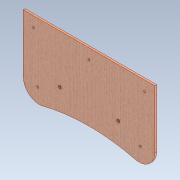
# Autodesk Inventor part: FTC Outside Panels
Saved by Autodesk Inventor 2020 (Build 240168000, 168)
## iProperties
Created: 2022-09-23
Part Number: FTC Outside Panels
Material: Wood (Oak)
Document SubType Name: Modeling
Designer: Jason
Density: 0.76 g/cm^3
Appearance: White Oak - Natural Medium Gloss
Author: Jason
Autodesk Inventor part; units mm, degrees
ref_plane "YZ Plane" through (0, 0, 0) normal (1, 0, 0) x (0, 1, 0)
ref_plane "XZ Plane" through (0, 0, 0) normal (0, 1, 0) x (-1, 0, 0)
ref_plane "XY Plane" through (0, 0, 0) normal (0, 0, 1) x (1, 0, 0)
sketch "Sketch1" plane through (0, 0, 0) normal (0, 0, 1) x (1, 0, 0)
  line L0 (49.2125, 0) -> (54.6328, 0)
  line L1 (357.1875, 0) -> (350.9902, 0)
  arc A0 (0, 49.2125) -> (65.0875, 2.6308) centre (49.2125, 49.2125) ccw
  arc A1 (345.2239, 1.4763) -> (406.4, 49.2125) centre (357.1875, 49.2125) ccw
  arc A2 (203.2, 19.05) -> (54.6328, 0) centre (202.8115, -566.7686) ccw
  arc A3 (350.9902, 0) -> (345.2239, 1.4763) centre (202.8115, -566.7686) ccw
  arc A4 (65.0875, 2.6308) -> (54.6328, 0) centre (202.8115, -566.7686) ccw
  arc A5 (350.9902, 0) -> (203.2, 19.05) centre (202.8115, -566.7686) ccw
  line L2 (0, 49.2125) -> (0, 228.6)
  line L3 (406.4, 228.6) -> (406.4, 49.2125)
  line L4 (0, 228.6) -> (406.4, 228.6)
  point P0 (0, 0)
  point P1 (57.0671, 0.6309)
  constraints: 16 point on circle, 10 end point, 6 centre point, 1 perpendicular, 1 vertical
extrude "Extrusion1" add sketch "Sketch1" along normal blind 5.5563 contours A0 L2 L4 L3 A1 A5 A2
sketch "Sketch2" plane through (0, 0, 5.5563) normal (0, 0, 1) x (1, 0, 0)
  arc A0 (0, 49.2125) -> (57.0671, 0.6309) centre (49.2125, 49.2125) ccw projected
  arc A1 (345.2239, 1.4763) -> (406.4, 49.2125) centre (357.1875, 49.2125) ccw projected
  line L0 (361.7622, 0.2131) -> (361.7412, 44.6631)
  line L1 (361.7412, 44.6631) -> (406.1912, 44.6631)
  line L2 (0.2109, 44.6609) -> (44.6609, 44.6609)
  line L3 (44.6609, 44.6609) -> (44.6609, 0.2109)
  line L4 (365.2681, 38.3131) -> (368.9342, 44.6631)
  line L5 (365.2681, 51.0131) -> (368.9342, 44.6631)
  line L6 (357.9357, 51.0131) -> (365.2681, 51.0131)
  line L7 (357.9357, 38.3131) -> (365.2681, 38.3131)
  line L8 (357.9357, 51.0131) -> (354.2695, 44.6631)
  line L9 (354.2695, 44.6631) -> (357.9357, 38.3131)
  line L10 (48.1878, 38.3109) -> (51.854, 44.6609)
  line L11 (48.1878, 51.0109) -> (51.854, 44.6609)
  line L12 (40.8554, 51.0109) -> (48.1878, 51.0109)
  line L13 (40.8554, 38.3109) -> (48.1878, 38.3109)
  line L14 (40.8554, 51.0109) -> (37.1893, 44.6609)
  line L15 (37.1893, 44.6609) -> (40.8554, 38.3109)
  circle A2 centre (361.7412, 44.6631) radius 2.9337
  circle A3 centre (44.6609, 44.6609) radius 2.9337
  point P0 (0, 0)
  dimension "d97" = 44.45
  dimension "d99" = 44.45
  dimension "d100" = 44.45
  dimension "d101" = 44.45
  dimension "d102" = 12.7
  dimension "d103" = 12.7
  dimension "d104" = 12.7
  dimension "d105" = 7.3323
  dimension "d106" = 7.3323
  dimension "d107" = 7.3323
  dimension "d108" = 7.3323
  dimension "d109" = 7.3323
  dimension "d110" = 7.3323
  dimension "d111" = 12.7
  dimension "d112" = 12.7
  dimension "d113" = 12.7
  dimension "d114" = 7.3323
  dimension "d115" = 7.3323
  dimension "d116" = 7.3323
  dimension "d117" = 7.3323
  dimension "d118" = 7.3323
  dimension "d119" = 7.3323
  dimension "d145" = 5.8674
  dimension "d156" = 5.8674
  constraints: 32 end point, 6 horizontal, 3 point on circle, 2 centre point, 2 coincident, 1 perpendicular
  measures "d97" distance of L0.end L0.start
  measures "d99" distance of L0.end L1.end
  measures "d100" distance of L2.start L2.end
  measures "d101" distance of L2.end L3.end
  measures "d102" distance between parallel lines of L5 L9
  measures "d103" distance between parallel lines of L8 L4
  measures "d104" distance between parallel lines of L6 L7
  measures "d105" distance of L8.start L8.end
  measures "d106" distance of L8.end L9.end
  measures "d107" distance of L7.end L4.end
  measures "d108" distance of L9.end L7.end
  measures "d109" distance of L5.start L4.end
  measures "d110" distance of L8.start L6.end
  measures "d111" distance between parallel lines of L11 L15
  measures "d112" distance between parallel lines of L14 L10
  measures "d113" distance between parallel lines of L12 L13
  measures "d114" distance of L14.start L14.end
  measures "d115" distance of L14.end L15.end
  measures "d116" distance of L13.end L10.end
  measures "d117" distance of L15.end L13.end
  measures "d118" distance of L11.start L10.end
  measures "d119" distance of L14.start L12.end
  measures "d145" diameter of A2
  measures "d156" diameter of A3
extrude "Extrusion2" cut sketch "Sketch2" against normal through all contours A3 L3 L2 | L2 L3 A3 | A2 L1 L0 | L0 L1 A2
sketch "Sketch5" plane through (-0.198, 12.7962, 5.5563) normal (0, 0, 1) x (1, 0, 0)
  circle A0 centre (31.948, 184.0538) radius 2.9337
  circle A1 centre (374.848, 184.0538) radius 2.9337
  line L0 (31.948, 184.0538) -> (203.398, 184.0538)
  circle A2 centre (203.398, 184.0538) radius 2.9337
  point P0 (0.198, 215.8038)
  dimension "d141" = 5.8674
  dimension "d140" = 5.8674
  dimension "d139" = 171.45
  dimension "d138" = 5.8674
  constraints: 3 centre point, 2 end point, 1 coincident, 1 horizontal
  measures "d141" diameter of A0
  measures "d140" diameter of A1
  measures "d139" distance of L0.start L0.end
  measures "d138" diameter of A2
extrude "Extrusion6" cut sketch "Sketch5" against normal up to surface (5.5563 mm away)
sketch "Sketch6" plane through (0, 0, 5.5563) normal (0, 0, 1) x (1, 0, 0)
  ellipse E0 centre (293.3334, 94.2801) end of major axis (293.3295, 96.2801) minor radius 2
  ellipse E1 centre (293.3643, 62.2802) end of major axis (293.3569, 64.2802) minor radius 2
  circle A0 centre (361.7412, 44.6631) radius 2.9337 projected
  line L0 (361.7412, 44.6631) -> (293.3643, 44.6631)
  line L1 (293.3643, 44.6631) -> (293.3643, 62.2802)
  ellipse E2 centre (113.007, 94.278) end of major axis (113.0032, 96.278) minor radius 2
  ellipse E3 centre (113.0379, 62.2781) end of major axis (113.0305, 64.2781) minor radius 2
  line L2 (113.0379, 44.6609) -> (113.0379, 62.2781)
  circle A1 centre (293.3643, 78.2802) radius 4.699
  circle A2 centre (113.0379, 78.278) radius 4.699
  circle A3 centre (44.6609, 44.6609) radius 2.9337 projected
  line L3 (44.6609, 44.6609) -> (113.0379, 44.6609)
  point P0 (0, 0)
  dimension "d147" = 17.6171
  dimension "d148" = 68.3769
  dimension "d150" = 17.6171
  dimension "d152" = 9.398
  dimension "d153" = 9.398
  dimension "d157" = 68.3769
  constraints: 8 end point, 2 centre point, 2 horizontal, 1 perpendicular, 1 vertical, 8 other
  measures "d147" distance of L0.end L1.end
  measures "d148" distance of L0.start L0.end
  measures "d150" distance of L2.start L2.end
  measures "d152" diameter of A1
  measures "d153" diameter of A2
  measures "d157" distance of L3.start L2.start
extrude "Extrusion7" cut sketch "Sketch6" against normal through all contours A1 | A2
body "Solid1"
